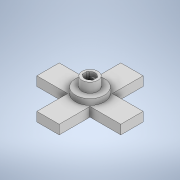
# Autodesk Inventor part: Motor_Key_Cross
Saved by Autodesk Inventor 2022 (Build 260153000, 153)
## iProperties
Created: 2023-03-24
Part Number: Motor_Key_Cross
Material: Generic
Document SubType Name: Modeling
Designer: zarek
Density: 1 g/cm^3
Appearance: Default
Author: zarek
Autodesk Inventor part; units mm, degrees
ref_plane "YZ Plane" through (0, 0, 0) normal (1, 0, 0) x (0, 1, 0)
ref_plane "XZ Plane" through (0, 0, 0) normal (0, 1, 0) x (-1, 0, 0)
ref_plane "XY Plane" through (0, 0, 0) normal (0, 0, 1) x (1, 0, 0)
sketch "Sketch1" plane through (0, 0, 0) normal (0, 1, 0) x (-1, 0, 0)
  line L0 (0, 0) -> (0, 25)
  line L1 (0, 0) -> (-25, 0)
  line L2 (0, 0) -> (0, -25)
  line L3 (0, 0) -> (25, 0)
  line L4 (25, 0) -> (25, -9)
  line L5 (0, -25) -> (9, -25)
  line L6 (9, -25) -> (9, -9)
  line L7 (9, -9) -> (25, -9)
  line L8 (0, -25) -> (-9, -25)
  line L9 (-9, -25) -> (-9, -9)
  line L10 (-9, -9) -> (-25, -9)
  line L11 (-25, -9) -> (-25, 0)
  line L12 (-25, 0) -> (-25, 9)
  line L13 (-25, 9) -> (-9, 9)
  line L14 (-9, 9) -> (-9, 25)
  line L15 (-9, 25) -> (0, 25)
  line L16 (9, 25) -> (0, 25)
  line L17 (9, 25) -> (9, 9)
  line L18 (9, 9) -> (25, 9)
  line L19 (25, 9) -> (25, 0)
  line L20 (21.8, -5.8) -> (5.8, -5.8)
  line L21 (5.8, -5.8) -> (5.8, -21.8)
  line L22 (5.8, -21.8) -> (-5.8, -21.8)
  line L23 (-5.8, -21.8) -> (-5.8, -5.8)
  line L24 (-5.8, -5.8) -> (-21.8, -5.8)
  line L25 (-21.8, -5.8) -> (-21.8, 5.8)
  line L26 (-21.8, 5.8) -> (-5.8, 5.8)
  line L27 (-5.8, 5.8) -> (-5.8, 21.8)
  line L28 (-5.8, 21.8) -> (5.8, 21.8)
  line L29 (5.8, 21.8) -> (5.8, 5.8)
  line L30 (5.8, 5.8) -> (21.8, 5.8)
  line L31 (21.8, 5.8) -> (21.8, -5.8)
  dimension "d0" = 25
  dimension "d1" = 25
  dimension "d2" = 25
  dimension "d3" = 25
  dimension "d4" = 9
  dimension "d5" = 9
  dimension "d6" = 9
  dimension "d7" = 9
  dimension "d8" = 9
  dimension "d9" = 9
  dimension "d10" = 9
  dimension "d11" = 9
  dimension "d34" = 3.2
  dimension "d35" = 3.2
  dimension "d36" = 3.2
  dimension "d37" = 3.2
  dimension "d38" = 3.2
  dimension "d39" = 3.2
  dimension "d40" = 3.2
  dimension "d41" = 3.2
  dimension "d42" = 3.2
  dimension "d43" = 3.2
  dimension "d44" = 3.2
  dimension "d45" = 3.2
  constraints: 64 end point, 17 perpendicular, 15 point on line, 4 horizontal, 2 vertical, 1 collinear
  measures "d0" distance of L0.start L0.end
  measures "d1" distance of L0.start L1.end
  measures "d2" distance of L0.start L2.end
  measures "d3" distance of L0.start L3.end
  measures "d4" distance of L3.end L4.end
  measures "d5" distance of L2.end L5.end
  measures "d6" distance of L2.end L8.end
  measures "d7" distance of L1.end L12.end
  measures "d8" distance between parallel lines of L3 L18
  measures "d9" distance between parallel lines of L0 L17
  measures "d10" distance between parallel lines of L14 L0
  measures "d11" distance between parallel lines of L10 L1
  measures "d34" distance between parallel lines of L20 L7
  measures "d35" distance between parallel lines of L4 L31
  measures "d36" distance between parallel lines of L18 L30
  measures "d37" distance between parallel lines of L29 L17
  measures "d38" distance between parallel lines of L16 L28
  measures "d39" distance between parallel lines of L14 L27
  measures "d40" distance between parallel lines of L13 L26
  measures "d41" distance between parallel lines of L11 L25
  measures "d42" distance between parallel lines of L24 L10
  measures "d43" distance between parallel lines of L23 L9
  measures "d44" distance between parallel lines of L22 L5
  measures "d45" distance between parallel lines of L6 L21
extrude "Extrusion1" add sketch "Sketch1" along normal blind 4.8 contours L1 L25 L26 L27 L28 L0 | L2 L22 L23 L24 L25 L1 | L3 L31 L20 L21 L22 L2 | L0 L28 L29 L30 L31 L3
sketch "Sketch3" plane through (0, 4.8, 0) normal (0, 1, 0) x (1, 0, 0)
  circle A0 centre (0, 0) radius 4.1
  dimension "d18" = 8.2
  constraints: 1 centre point, 1 coincident
  measures "d18" diameter of A0
extrude "Extrusion3" add sketch "Sketch3" along normal blind 8
sketch "Sketch6" plane through (0, 4.8, 0) normal (0, 1, 0) x (1, 0, 0)
  circle A0 centre (0, 0) radius 7.5
  dimension "d31" = 15
  constraints: 1 centre point, 1 coincident
  measures "d31" diameter of A0
extrude "Extrusion6" add sketch "Sketch6" along normal blind 3
sketch "Sketch4" plane through (0, 12.8, 0) normal (0, 1, 0) x (1, 0, 0)
  line L0 (-0.0005, -0.0003) -> (-0.0005, -1.7003)
  line L1 (-0.0005, -1.7003) -> (2.6995, -1.7003)
  line L2 (2.6995, -1.7003) -> (2.6995, 1.6997)
  line L3 (2.6995, 1.6997) -> (-2.7005, 1.6997)
  line L4 (-2.7005, 1.6997) -> (-2.7005, -1.7003)
  line L5 (-2.7005, -1.7003) -> (-0.0005, -1.7003)
  point P0 (0, 0)
  dimension "d21" = 1.7
  dimension "d22" = 2.7
  dimension "d23" = 3.4
  dimension "d24" = 5.4
  constraints: 12 end point, 5 perpendicular, 1 point on line, 1 vertical
  measures "d21" distance of L0.start L0.end
  measures "d22" distance of L0.end L1.end
  measures "d23" distance of L1.end L2.end
  measures "d24" distance of L2.end L3.end
extrude "Extrusion4" cut sketch "Sketch4" against normal blind 8.2
sketch "Sketch5" plane through (0, 12.8, 0) normal (0, 1, 0) x (1, 0, 0)
  circle A0 centre (0, 0) radius 2.7
  dimension "d27" = 5.4
  constraints: 1 centre point, 1 coincident
  measures "d27" diameter of A0
extrude "Extrusion5" cut sketch "Sketch5" against normal blind 2.2
fillet "Fillet1" radius 0.635 4 edges at (-2.7005, 8.7, -1.6997) (-2.7005, 8.7, 1.7003) (2.6995, 8.7, -1.6997) (2.6995, 8.7, 1.7003)
equation "\"d5\" = d4"
equation "\"d6\" = d4"
equation "\"d7\" = d4"
equation "\"d35\" = d34"
equation "\"d36\" = d34"
equation "\"d37\" = d34"
equation "\"d38\" = d34"
equation "\"d39\" = d34"
equation "\"d40\" = d34"
equation "\"d41\" = d34"
equation "\"d42\" = d34"
equation "\"d44\" = d34"
equation "\"d21\" = 0.5 * d23"
body "Solid1"
